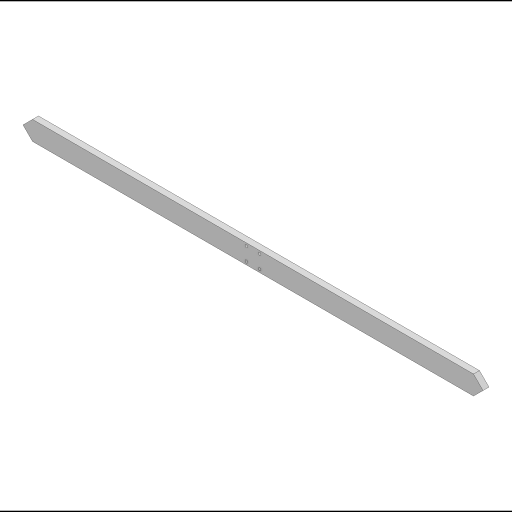
# Autodesk Inventor part: Motor Strap 5-16
Saved by Autodesk Inventor 2023 (Build 270158000, 158)
## iProperties
Created: 2022-10-29
Part Number: Motor Strap 5-16
Material: Generic
Document SubType Name: Modeling
Designer: kamer
Density: 1 g/cm^3
Appearance: Default
Author: kamer
Autodesk Inventor part; units mm, degrees
ref_plane "YZ Plane" through (0, 0, 0) normal (1, 0, 0) x (0, 1, 0)
ref_plane "XZ Plane" through (0, 0, 0) normal (0, 1, 0) x (-1, 0, 0)
ref_plane "XY Plane" through (0, 0, 0) normal (0, 0, 1) x (1, 0, 0)
sketch "Sketch1" plane through (0, 0, 0) normal (0, 0, 1) x (1, 0, 0)
  line L0 (0, 0) -> (12.7, 12.7)
  line L1 (0, 0) -> (12.7, -12.7)
  line L2 (12.7, -12.7) -> (600.1258, -12.7)
  line L3 (600.1258, -12.7) -> (612.8258, 0)
  line L4 (612.8258, 0) -> (600.1258, 12.7)
  line L5 (600.1258, 12.7) -> (12.7, 12.7)
  line L6 (0, 0) -> (26.9875, 0) construction
  dimension "d0" = 90
  dimension "d1" = 45
  dimension "d2" = 612.8258
  dimension "d3" = 25.4
  dimension "d4" = 12.7
  dimension "d5" = 0
  constraints: 14 end point, 2 horizontal, 2 perpendicular, 1 parallel
  measures "d0" angle of L1 L0
  measures "d1" angle of L0 L6
  measures "d2" distance of L3.end L0.start
  measures "d3" distance between parallel lines of L2 L5
  measures "d4" distance between parallel lines of L5 L6
  measures "d5" horizontal distance of L4.end L2.end
extrude "Extrusion1" add sketch "Sketch1" along normal blind 7.9375
sketch "Sketch2" plane through (0, 0, 7.9375) normal (0, 0, 1) x (1, 0, 0)
  line L0 (12.7, 12.7) -> (0, 0) construction
  line L1 (0, 0) -> (306.4129, 0) construction
  line L2 (600.1258, 12.7) -> (12.7, 12.7) construction
  line L3 (306.4129, 0) -> (306.4129, 138.1125) construction
  circle A0 centre (306.4129, 0) radius 12.5 construction
  line L4 (297.5741, 8.8388) -> (315.2517, 8.8388) construction
  line L5 (315.2517, 8.8388) -> (315.2517, -8.8388) construction
  line L6 (315.2517, -8.8388) -> (297.5741, -8.8388) construction
  line L7 (297.5741, -8.8388) -> (297.5741, 8.8388) construction
  circle A1 centre (297.5741, 8.8388) radius 1.75
  circle A2 centre (315.2517, 8.8388) radius 1.75
  circle A3 centre (315.2517, -8.8388) radius 1.75
  circle A4 centre (297.5741, -8.8388) radius 1.75
  dimension "d8" = 306.4129
  dimension "d9" = 25
  dimension "d10" = 3.5
  dimension "d11" = 3.5
  dimension "d12" = 3.5
  dimension "d13" = 3.5
  constraints: 12 end point, 5 centre point, 5 coincident, 3 parallel, 3 perpendicular, 3 point on circle, 1 horizontal
  measures "d8" distance of L1.end L0.end
  measures "d9" diameter of A0
  measures "d10" diameter of A1
  measures "d11" diameter of A2
  measures "d12" diameter of A3
  measures "d13" diameter of A4
extrude "Extrusion2" cut sketch "Sketch2" against normal through all
body "Solid1"
